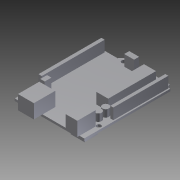
# Autodesk Inventor part: Arduino
Saved by Autodesk Inventor 2011 SP2 (Build 150309200, 309)
## iProperties
Created: 2015-01-24
Part Number: Arduino
Document SubType Name: Modeling
Designer: Ernest
Density: 1 g/cm^3
Mass: 15.9204 g
Surface Area: 125.226 cm^2
Volume: 15.9204 cm^3
Author: Ernest
Autodesk Inventor part; units mm, degrees
ref_plane "YZ Plane" through (0, 0, 0) normal (1, 0, 0) x (0, 1, 0)
ref_plane "XZ Plane" through (0, 0, 0) normal (0, 1, 0) x (-1, 0, 0)
ref_plane "XY Plane" through (0, 0, 0) normal (0, 0, 1) x (1, 0, 0)
sketch "Sketch1" plane through (0, 0, 0) normal (0, 0, 1) x (1, 0, 0)
  line L0 (0, 0) -> (68.9, 0)
  line L1 (68.9, 0) -> (68.9, 1.7)
  line L2 (68.9, 1.7) -> (0, 1.7)
  line L3 (0, 1.7) -> (0, 0)
  dimension "d0" = 68.9
  dimension "d1" = 1.7
  constraints: 8 end point, 2 parallel, 1 horizontal, 1 perpendicular
  measures "d0" distance of L2.end L1.end
  measures "d1" distance between parallel lines of L0 L2
extrude "Extrusion1" add sketch "Sketch1" along normal blind 53.3
sketch "Sketch2" plane through (0, 1.7, 0) normal (0, 1, 0) x (1, 0, 0)
  line L0 (0, -53.3) -> (68.9, -53.3) projected
  line L1 (68.9, 0) -> (68.9, -53.3) projected
  line L2 (68.9, 0) -> (0, 0) projected
  line L3 (0, 0) -> (0, -53.3) projected
  line L4 (66.2, 0) -> (66.2, -53.3)
  line L5 (68.9, -53.3) -> (0, -53.3) projected
  circle A0 centre (66.25, -47.55) radius 1.65
  circle A1 centre (66.25, -17.45) radius 1.65
  circle A2 centre (13.8, -2.65) radius 1.65
  circle A3 centre (13.95, -50.65) radius 1.65
  line L6 (66.2, 0) -> (66.2, -12.7)
  line L7 (66.2, -12.7) -> (68.9, -15.2036)
  line L8 (68.9, 0) -> (68.9, -15.2036)
  line L9 (68.9, 0) -> (68.9, -53.3) projected
  line L10 (66.2, 0) -> (68.9, 0)
  line L11 (0, 0) -> (68.9, 0) projected
  line L12 (68.9, 0) -> (66.2, 0)
  line L13 (66.2, -53.3) -> (66.2, -51.5)
  line L14 (66.2, -51.5) -> (68.9, -49.9641)
  line L15 (68.9, -53.3) -> (66.2, -53.3)
  line L16 (68.9, -53.3) -> (68.9, -49.9641)
  dimension "d4" = 2.7
  dimension "d5" = 5.75
  dimension "d6" = 1
  dimension "d7" = 3.3
  dimension "d8" = 3.3
  dimension "d9" = 3.3
  dimension "d10" = 3.3
  dimension "d11" = 15.8
  dimension "d12" = 1
  dimension "d13" = 1
  dimension "d14" = 1
  dimension "d15" = 13.8
  dimension "d16" = 12.3
  dimension "d17" = 12.7
  dimension "d18" = 2.5036
  dimension "d19" = 1.8
  dimension "d20" = 1.5359
  constraints: 20 end point, 6 point on line, 4 centre point, 4 collinear, 2 perpendicular
  measures "d4" distance between parallel lines of L1 L4
  measures "d5" distance from line of A0.centre L0
  measures "d6" distance edge to line of A0 L1
  measures "d7" diameter of A0
  measures "d8" diameter of A1
  measures "d9" diameter of A2
  measures "d10" diameter of A3
  measures "d11" distance edge to line of A1 L2
  measures "d12" distance edge to line of A1 L1
  measures "d13" distance edge to line of A2 L2
  measures "d14" distance edge to line of A3 L0
  measures "d15" distance from line of A2.centre L3
  measures "d16" distance edge to line of A3 L3
  measures "d17" distance of L4.start L6.end
  measures "d18" vertical distance of L6.end L7.end
  measures "d19" distance of L4.end L13.end
  measures "d20" vertical distance of L13.end L14.end
extrude "Extrusion2" cut sketch "Sketch2" against normal blind 53.3 contours L4 L14 L1 L0 | L2 L1 L7 L4 | A0 L4 | L4 A0 | A1 L4 | L4 A1 | A2 | A3
sketch "Sketch3" plane through (0, 1.7, 53.3) normal (0, 1, 0) x (1, 0, 0)
  line L0 (66.2, 53.3) -> (0, 53.3) projected
  line L1 (0, 53.3) -> (0, 0) projected
  line L2 (0, 0) -> (66.2, 0) projected
  line L3 (9.75, 44.2) -> (-6.65, 44.2)
  line L4 (-6.65, 44.2) -> (-6.65, 32)
  line L5 (-6.65, 32) -> (9.75, 32)
  line L6 (9.75, 32) -> (9.75, 44.2)
  line L7 (12.3, 12.4) -> (-1.7, 12.4)
  line L8 (-1.7, 12.4) -> (-1.7, 3.6)
  line L9 (-1.7, 3.6) -> (12.3, 3.6)
  line L10 (12.3, 3.6) -> (12.3, 12.4)
  dimension "d23" = 9.1
  dimension "d24" = 9.75
  dimension "d25" = 16.4
  dimension "d26" = 12.2
  dimension "d27" = 8.8
  dimension "d28" = 14
  dimension "d29" = 12.4
  dimension "d30" = 1.7
  constraints: 16 end point, 4 parallel, 2 horizontal, 2 perpendicular
  measures "d23" distance between parallel lines of L3 L0
  measures "d24" distance between parallel lines of L6 L1
  measures "d25" distance of L4.end L5.end
  measures "d26" distance of L5.end L3.start
  measures "d27" distance of L7.end L8.end
  measures "d28" distance of L7.start L7.end
  measures "d29" distance between parallel lines of L2 L7
  measures "d30" distance between parallel lines of L1 L8
extrude "Extrusion3" add sketch "Sketch3" along normal blind 10.8
sketch "Sketch4" plane through (0, 0, 0) normal (0, -1, 0) x (1, 0, 0)
  line L0 (1.7559, 51.8193) -> (11.7504, 51.8193)
  line L1 (11.7504, 51.8193) -> (11.7504, 41.2908)
  line L2 (11.7504, 41.2908) -> (1.7559, 41.2908)
  line L3 (1.7559, 41.2908) -> (1.7559, 51.8193)
  line L4 (2.8536, 9.1407) -> (9.75, 9.1407)
  line L5 (9.75, 9.1407) -> (9.75, 23.0608)
  line L6 (9.75, 23.0608) -> (2.8536, 23.0608)
  line L7 (2.8536, 23.0608) -> (2.8536, 9.1407)
  line L8 (17.3733, 1) -> (64.6, 1)
  line L9 (64.6, 1) -> (64.6, 3.3066)
  line L10 (64.6, 3.3066) -> (17.3733, 3.3066)
  line L11 (17.3733, 3.3066) -> (17.3733, 1)
  line L12 (14.8067, 10.5642) -> (19.5461, 10.5642)
  line L13 (19.5461, 10.5642) -> (19.5461, 5.2627)
  line L14 (19.5461, 5.2627) -> (14.8067, 5.2627)
  line L15 (14.8067, 5.2627) -> (14.8067, 10.5642)
  line L16 (23.3828, 51.8193) -> (64.9232, 51.8193)
  line L17 (64.9232, 51.8193) -> (64.9232, 49.9641)
  line L18 (64.9232, 49.9641) -> (23.3828, 49.9641)
  line L19 (23.3828, 49.9641) -> (23.3828, 51.8193)
  line L20 (63.5698, 43.7351) -> (27.6508, 43.7351)
  line L21 (27.6508, 43.7351) -> (27.6508, 41.2908)
  line L22 (27.6508, 41.2908) -> (63.5698, 41.2908)
  line L23 (63.5698, 41.2908) -> (63.5698, 43.7351)
  line L24 (63.5698, 37.8841) -> (27.6508, 37.8841)
  line L25 (27.6508, 37.8841) -> (27.6508, 35.2553)
  line L26 (27.6508, 35.2553) -> (63.5698, 35.2553)
  line L27 (63.5698, 35.2553) -> (63.5698, 37.8841)
  line L28 (63.1531, 29.6705) -> (67.0258, 29.6705)
  line L29 (67.0258, 29.6705) -> (67.0258, 20.8923)
  line L30 (67.0258, 20.8923) -> (63.1531, 20.8923)
  line L31 (63.1531, 20.8923) -> (63.1531, 29.6705)
  constraints: 64 end point, 16 parallel, 8 horizontal, 8 perpendicular
extrude "Extrusion5" add sketch "Sketch4" along normal blind 1.2 contours L11 L10 L9 L8 | L12 L13 L14 L15 | L16 L17 L18 L19 | L23 L22 L21 L20 | L27 L26 L25 L24 | L28 L29 L30 L31
extrude "Extrusion6" add sketch "Sketch4" along normal blind 2.4 contours L0 L1 L2 L3 | L7 L6 L5 L4
sketch "Sketch5" plane through (0, 1.7, 0) normal (0, 1, 0) x (1, 0, 0)
  line L0 (16.8373, -1.3594) -> (65.158, -1.3594)
  line L1 (65.158, -1.3594) -> (65.158, -3.8941)
  line L2 (65.158, -3.8941) -> (16.8373, -3.8941)
  line L3 (16.8373, -3.8941) -> (16.8373, -1.3594)
  line L4 (14.3267, -5.2627) -> (19.5222, -5.2627)
  line L5 (19.5222, -5.2627) -> (19.5222, -8.6683)
  line L6 (19.5222, -8.6683) -> (14.3267, -8.6683)
  line L7 (14.3267, -8.6683) -> (14.3267, -5.2627)
  line L8 (67.0258, -29.6705) -> (67.0258, -20.8923) projected
  line L9 (63.1531, -20.8923) -> (67.0258, -20.8923)
  line L10 (67.0258, -20.8923) -> (67.0258, -28.4607)
  line L11 (67.0258, -28.4607) -> (63.1531, -28.4607)
  line L12 (63.1531, -28.4607) -> (63.1531, -20.8923)
  line L13 (23.3828, -52.3) -> (65.6017, -52.3)
  line L14 (65.6017, -52.3) -> (65.6017, -49.9641)
  line L15 (65.6017, -49.9641) -> (23.3828, -49.9641)
  line L16 (23.3828, -49.9641) -> (23.3828, -52.3)
  line L17 (27.2824, -35.2553) -> (63.9894, -35.2553)
  line L18 (63.9894, -35.2553) -> (63.9894, -44.4726)
  line L19 (63.9894, -44.4726) -> (27.2824, -44.4726)
  line L20 (27.2824, -44.4726) -> (27.2824, -35.2553)
  circle A0 centre (23.9092, -45.9) radius 2.5569
  circle A1 centre (18.2181, -45.9) radius 2.5569
  constraints: 40 end point, 10 parallel, 5 horizontal, 5 perpendicular, 2 centre point, 1 point on line
extrude "Extrusion7" add sketch "Sketch5" along normal blind 8.4 contours L0 L1 L2 L3 | L4 L5 L6 L7 | L11 L12 L9 L8 | L16 L15 L14 L13 | L17 L18 L19 L20
extrude "Extrusion8" add sketch "Sketch5" along normal blind 5.6 contours A0 | A1
body "Solid1"
